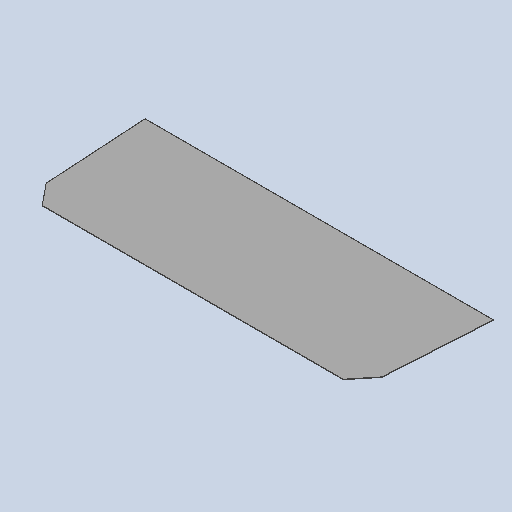
# Autodesk Inventor part: MSC 075 face 2
Saved by Autodesk Inventor 2025 (Build 290162010, 162A)
## iProperties
Created: 2024-06-16
Part Number: MSC 075 face 2
Material: AISI304
Document SubType Name: Sheet Metal
Designer: admin
Density: 8 g/cm^3
Sheet Metal Rule: AISI304 2mm Die16
Appearance: Default
Stock Number: МОО 075 морда 2
Flat Pattern Width: 57.4993 cm
Flat Pattern Length: 158.32 cm
Flat Pattern Area: 9103.28 cm^2
Sheet Metal Width: 574,993 mm
Sheet Metal Length: 1583,197 mm
Sheet Metal Area: 910328,018 mm^2
Author: admin
Autodesk Inventor part; units mm, degrees
ref_plane "YZ Plane" through (0, 0, 0) normal (1, 0, 0) x (0, 1, 0)
ref_plane "XZ Plane" through (0, 0, 0) normal (0, 1, 0) x (-1, 0, 0)
ref_plane "XY Plane" through (0, 0, 0) normal (0, 0, 1) x (1, 0, 0)
sketch "Sketch1" plane through (0, 0, 0) normal (0, 0, 1) x (1, 0, 0)
  line L0 (791.5986, 0) -> (791.5986, -574.9935) construction
  line L1 (791.5986, -574.9935) -> (0, -574.9935)
  line L2 (751.2327, -476.7052) -> (671.2185, -574.9935) construction
  ellipse E0 centre (-10250, 897.8357) end of major axis (-10250, -13530.831) minor radius 11053 (753.0938, -471.7446) -> (781.5803, 0) ccw construction
  line L3 (791.5986, 0) -> (762.7071, -478.4497)
  line L4 (684.1131, -574.9935) -> (791.5986, -442.9599)
  line L5 (753.0938, -471.7446) -> (763.0756, -472.3473) construction
  line L6 (781.5803, 0) -> (791.5622, -0.6028) construction
  line L7 (0, -574.9935) -> (0, 0)
  line L8 (0, 0) -> (791.5986, 0)
  dimension "d3" = 10
  dimension "d4" = 10
  dimension "d5" = 10
  measures "d3" distance between parallel lines of L4 L2
  measures "d4" distance of L5.start L5.end
  measures "d5" distance of L6.start L6.end
extrude "Plate1" add sketch "Sketch1" along normal blind 2
mirror "Mirror1" about plane through (0, 0, 0) normal (1, 0, 0) of "Plate1"
equation "\"d2\" = Thickness"
equation "\"BendReliefWidth\" = Thickness"
equation "\"BendReliefDepth\" = 0.5 * Thickness"
equation "\"CornerReliefSize\" = 4 * Thickness"
equation "\"MinimumRemnant\" = 2 * Thickness"
equation "\"TransitionRadius\" = BendRadius"
equation "\"JacobiRadiusSize\" = BendRadius"
equation "\"GapSize\" = Thickness"
equation "\"Thickness\" = 2"
equation "\"BendRadius\" = 2.75"
body "Solid1"
